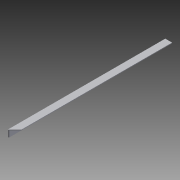
# Autodesk Inventor part: Aluminum Angle 3 Left
Saved by Autodesk Inventor 2014 (Build 180170000, 170)
## iProperties
Created: 2014-02-02
Part Number: Aluminum Angle 3 Left
Material: Aluminum 6061
Document SubType Name: Modeling
Designer: Andrew Toennies
Mass: 18.3798 g
Surface Area: 113.157 cm^2
Volume: 6.7822 cm^3
Density: 2.71 g/cm^3
Appearance: Aluminum - Flat
Author: Andrew Toennies
Autodesk Inventor part; units mm, degrees
ref_plane "YZ Plane" through (0, 0, 0) normal (1, 0, 0) x (0, 1, 0)
ref_plane "XZ Plane" through (0, 0, 0) normal (0, 1, 0) x (-1, 0, 0)
ref_plane "XY Plane" through (0, 0, 0) normal (0, 0, 1) x (1, 0, 0)
sketch "Sketch1" plane through (0, 0, 0) normal (0, 0, 1) x (1, 0, 0)
  line L0 (0, 0) -> (0, 12.7)
  line L1 (0, 12.7) -> (12.7, 12.7)
  line L2 (12.7, 12.7) -> (12.7, 11.43)
  line L3 (12.7, 11.43) -> (1.27, 11.43)
  line L4 (1.27, 11.43) -> (1.27, 0)
  line L5 (1.27, 0) -> (0, 0)
  dimension "d0" = 12.7
  dimension "d1" = 12.7
  dimension "d2" = 1.27
  dimension "d3" = 11.43
  constraints: 12 end point, 4 parallel, 1 perpendicular, 1 vertical
  measures "d0" distance of L0.start L0.end
  measures "d1" distance of L0.end L1.end
  measures "d2" distance of L1.end L2.end
  measures "d3" distance of L2.end L3.end
extrude "Extrusion1" add sketch "Sketch1" along normal blind 292.1
sketch "Sketch3" plane through (0, 12.7, 0) normal (0, 1, 0) x (1, 0, 0)
  line L0 (12.7, -292.1) -> (0, -292.1) projected
  line L1 (12.7, 0) -> (12.7, -292.1) projected
  line L2 (0, -292.1) -> (12.7, -279.4)
  dimension "d10" = 45
  constraints: 2 end point, 1 point on line
  measures "d10" angle of L0 L2
extrude "Extrusion3" cut sketch "Sketch3" against normal blind 25.4
body "Solid1"
